Autodesk Fusion 360 part; units mm, degrees
(part 8 of 15)
  spline S126 degree 5 poles (-18.825, -121.4416) (-18.8248, -121.4521) (-18.824, -121.4806) (-18.8228, -121.5269) (-18.8208, -121.5911) (-18.818, -121.6733) (-18.8145, -121.7628) (-18.8106, -121.8524) (-18.8063, -121.942) (-18.8015, -122.0317) (-18.7964, -122.1214) (-18.7909, -122.2111) (-18.785, -122.3009) (-18.7788, -122.3908) (-18.7721, -122.4807) (-18.7651, -122.5706) (-18.7577, -122.6606) (-18.7499, -122.7506) (-18.7418, -122.8406) (-18.7333, -122.9307) (-18.7245, -123.0208) (-18.7153, -123.111) (-18.7057, -123.2012) (-18.6959, -123.2914) (-18.6856, -123.3816) (-18.6751, -123.4719) (-18.6641, -123.5622) (-18.6529, -123.6525) (-18.6413, -123.7428) (-18.6294, -123.8332) (-18.6172, -123.9236) (-18.6046, -124.014) (-18.5918, -124.1045) (-18.5786, -124.1949) (-18.565, -124.2854) (-18.5512, -124.3759) (-18.537, -124.4664) (-18.5226, -124.557) (-18.5078, -124.6475) (-18.4927, -124.7381) (-18.4774, -124.8287) (-18.4617, -124.9193) (-18.4457, -125.0099) (-18.4326, -125.0824) (-18.4227, -125.1368) (-18.4161, -125.1731) (-18.4127, -125.1912) knots 0.405839 0.405839 0.405839 0.405839 0.405839 0.405839 0.414286 0.428571 0.442857 0.457143 0.471429 0.485714 0.5 0.514286 0.528571 0.542857 0.557143 0.571429 0.585714 0.6 0.614286 0.628571 0.642857 0.657143 0.671429 0.685714 0.7 0.714286 0.728571 0.742857 0.757143 0.771429 0.785714 0.8 0.814286 0.828571 0.842857 0.857143 0.871429 0.885714 0.9 0.914286 0.928571 0.942857 0.957143 0.971429 0.985714 1 1 1 1 1 1
  arc A127 (-18.4127, -125.1912) -> (-17.1202, -125.4724) centre (-2.0032, -52.8695) ccw
  spline S127 degree 5 poles (-17.1202, -125.4724) (-17.1096, -125.4573) (-17.0884, -125.4271) (-17.0568, -125.3817) (-17.0149, -125.3212) (-16.9627, -125.2454) (-16.9108, -125.1695) (-16.8591, -125.0935) (-16.8078, -125.0174) (-16.7567, -124.9411) (-16.706, -124.8648) (-16.6555, -124.7883) (-16.6053, -124.7117) (-16.5554, -124.635) (-16.5058, -124.5582) (-16.4565, -124.4813) (-16.4076, -124.4043) (-16.3589, -124.3271) (-16.3105, -124.2499) (-16.2624, -124.1725) (-16.2147, -124.095) (-16.1673, -124.0174) (-16.1202, -123.9397) (-16.0734, -123.8618) (-16.0269, -123.7839) (-15.9808, -123.7058) (-15.9349, -123.6277) (-15.8895, -123.5494) (-15.8443, -123.4709) (-15.7995, -123.3924) (-15.7551, -123.3138) (-15.711, -123.235) (-15.6672, -123.1561) (-15.6238, -123.0771) (-15.5808, -122.998) (-15.5381, -122.9187) (-15.4958, -122.8394) (-15.4539, -122.7599) (-15.4124, -122.6803) (-15.3712, -122.6005) (-15.3305, -122.5207) (-15.2901, -122.4407) (-15.2534, -122.3672) (-15.2249, -122.3096) (-15.2045, -122.2679) (-15.1921, -122.2424) (-15.1874, -122.2329) knots -1 -1 -1 -1 -1 -1 -0.985714 -0.971429 -0.957143 -0.942857 -0.928571 -0.914286 -0.9 -0.885714 -0.871429 -0.857143 -0.842857 -0.828571 -0.814286 -0.8 -0.785714 -0.771429 -0.757143 -0.742857 -0.728571 -0.714286 -0.7 -0.685714 -0.671429 -0.657143 -0.642857 -0.628571 -0.614286 -0.6 -0.585714 -0.571429 -0.557143 -0.542857 -0.528571 -0.514286 -0.5 -0.485714 -0.471429 -0.457143 -0.442857 -0.428571 -0.414286 -0.405839 -0.405839 -0.405839 -0.405839 -0.405839 -0.405839
  arc A128 (-15.1874, -122.2329) -> (-13.8903, -122.4669) centre (-2.0032, -52.8695) ccw
  spline S128 degree 5 poles (-13.8903, -122.4669) (-13.8893, -122.4774) (-13.8865, -122.5057) (-13.882, -122.5519) (-13.8754, -122.6158) (-13.8667, -122.6975) (-13.8569, -122.7866) (-13.8466, -122.8756) (-13.8359, -122.9647) (-13.8248, -123.0538) (-13.8133, -123.1429) (-13.8014, -123.2321) (-13.7891, -123.3212) (-13.7764, -123.4104) (-13.7634, -123.4996) (-13.7499, -123.5888) (-13.7362, -123.678) (-13.722, -123.7672) (-13.7075, -123.8565) (-13.6926, -123.9457) (-13.6773, -124.035) (-13.6617, -124.1242) (-13.6458, -124.2135) (-13.6295, -124.3028) (-13.6128, -124.3921) (-13.5959, -124.4813) (-13.5785, -124.5706) (-13.5609, -124.6599) (-13.5429, -124.7492) (-13.5246, -124.8385) (-13.5059, -124.9278) (-13.4869, -125.0171) (-13.4676, -125.1064) (-13.448, -125.1957) (-13.4281, -125.285) (-13.4078, -125.3742) (-13.3873, -125.4635) (-13.3664, -125.5528) (-13.3452, -125.6421) (-13.3237, -125.7314) (-13.3019, -125.8206) (-13.2798, -125.9099) (-13.2573, -125.9991) (-13.2392, -126.0705) (-13.2254, -126.1241) (-13.2162, -126.1597) (-13.2115, -126.1776) knots 0.405839 0.405839 0.405839 0.405839 0.405839 0.405839 0.414286 0.428571 0.442857 0.457143 0.471429 0.485714 0.5 0.514286 0.528571 0.542857 0.557143 0.571429 0.585714 0.6 0.614286 0.628571 0.642857 0.657143 0.671429 0.685714 0.7 0.714286 0.728571 0.742857 0.757143 0.771429 0.785714 0.8 0.814286 0.828571 0.842857 0.857143 0.871429 0.885714 0.9 0.914286 0.928571 0.942857 0.957143 0.971429 0.985714 1 1 1 1 1 1
  arc A129 (-13.2115, -126.1776) -> (-11.9022, -126.3658) centre (-2.0032, -52.8695) ccw
  spline S129 degree 5 poles (-11.9022, -126.3658) (-11.8927, -126.35) (-11.8738, -126.3184) (-11.8455, -126.2709) (-11.808, -126.2075) (-11.7613, -126.1282) (-11.7149, -126.0488) (-11.6689, -125.9693) (-11.6231, -125.8897) (-11.5776, -125.81) (-11.5324, -125.7302) (-11.4875, -125.6503) (-11.4429, -125.5704) (-11.3986, -125.4903) (-11.3547, -125.4102) (-11.311, -125.3299) (-11.2676, -125.2496) (-11.2246, -125.1692) (-11.1818, -125.0887) (-11.1394, -125.0081) (-11.0973, -124.9274) (-11.0555, -124.8466) (-11.0141, -124.7657) (-10.973, -124.6847) (-10.9322, -124.6037) (-10.8917, -124.5225) (-10.8516, -124.4412) (-10.8118, -124.3599) (-10.7724, -124.2785) (-10.7333, -124.1969) (-10.6946, -124.1153) (-10.6562, -124.0336) (-10.6182, -123.9518) (-10.5806, -123.8699) (-10.5433, -123.7879) (-10.5064, -123.7058) (-10.4699, -123.6236) (-10.4337, -123.5414) (-10.398, -123.459) (-10.3626, -123.3765) (-10.3276, -123.294) (-10.2931, -123.2113) (-10.2617, -123.1353) (-10.2374, -123.0759) (-10.2201, -123.0329) (-10.2095, -123.0065) (-10.2055, -122.9967) knots -1 -1 -1 -1 -1 -1 -0.985714 -0.971429 -0.957143 -0.942857 -0.928571 -0.914286 -0.9 -0.885714 -0.871429 -0.857143 -0.842857 -0.828571 -0.814286 -0.8 -0.785714 -0.771429 -0.757143 -0.742857 -0.728571 -0.714286 -0.7 -0.685714 -0.671429 -0.657143 -0.642857 -0.628571 -0.614286 -0.6 -0.585714 -0.571429 -0.557143 -0.542857 -0.528571 -0.514286 -0.5 -0.485714 -0.471429 -0.457143 -0.442857 -0.428571 -0.414286 -0.405839 -0.405839 -0.405839 -0.405839 -0.405839 -0.405839
  arc A130 (-10.2055, -122.9967) -> (-8.895, -123.1376) centre (-2.0032, -52.8695) ccw
  spline S130 degree 5 poles (-8.895, -123.1376) (-8.8932, -123.148) (-8.8884, -123.1761) (-8.8806, -123.2217) (-8.8695, -123.285) (-8.855, -123.3659) (-8.8388, -123.454) (-8.8222, -123.5421) (-8.8052, -123.6302) (-8.7878, -123.7183) (-8.7699, -123.8064) (-8.7517, -123.8945) (-8.7331, -123.9825) (-8.7141, -124.0706) (-8.6947, -124.1586) (-8.675, -124.2466) (-8.6548, -124.3346) (-8.6343, -124.4226) (-8.6135, -124.5106) (-8.5923, -124.5985) (-8.5707, -124.6865) (-8.5488, -124.7744) (-8.5265, -124.8623) (-8.5039, -124.9502) (-8.4809, -125.038) (-8.4576, -125.1259) (-8.4339, -125.2137) (-8.41, -125.3015) (-8.3856, -125.3893) (-8.361, -125.4771) (-8.336, -125.5648) (-8.3107, -125.6525) (-8.2851, -125.7402) (-8.2592, -125.8279) (-8.2329, -125.9155) (-8.2063, -126.0031) (-8.1794, -126.0907) (-8.1522, -126.1783) (-8.1247, -126.2658) (-8.0969, -126.3533) (-8.0688, -126.4408) (-8.0404, -126.5282) (-8.0117, -126.6157) (-7.9884, -126.6856) (-7.9709, -126.738) (-7.9591, -126.7729) (-7.9532, -126.7904) knots 0.405839 0.405839 0.405839 0.405839 0.405839 0.405839 0.414286 0.428571 0.442857 0.457143 0.471429 0.485714 0.5 0.514286 0.528571 0.542857 0.557143 0.571429 0.585714 0.6 0.614286 0.628571 0.642857 0.657143 0.671429 0.685714 0.7 0.714286 0.728571 0.742857 0.757143 0.771429 0.785714 0.8 0.814286 0.828571 0.842857 0.857143 0.871429 0.885714 0.9 0.914286 0.928571 0.942857 0.957143 0.971429 0.985714 1 1 1 1 1 1
  arc A131 (-7.9532, -126.7904) -> (-6.6338, -126.8848) centre (-2.0032, -52.8695) ccw
  spline S131 degree 5 poles (-6.6338, -126.8848) (-6.6255, -126.8683) (-6.6089, -126.8354) (-6.584, -126.786) (-6.5511, -126.7201) (-6.5102, -126.6377) (-6.4697, -126.5552) (-6.4294, -126.4726) (-6.3894, -126.3899) (-6.3497, -126.3072) (-6.3103, -126.2244) (-6.2712, -126.1415) (-6.2325, -126.0586) (-6.194, -125.9756) (-6.1558, -125.8925) (-6.118, -125.8093) (-6.0805, -125.7261) (-6.0433, -125.6428) (-6.0064, -125.5595) (-5.9698, -125.476) (-5.9336, -125.3925) (-5.8977, -125.309) (-5.8621, -125.2253) (-5.8269, -125.1416) (-5.792, -125.0579) (-5.7574, -124.974) (-5.7232, -124.8901) (-5.6893, -124.8062) (-5.6558, -124.7221) (-5.6227, -124.638) (-5.5898, -124.5538) (-5.5574, -124.4696) (-5.5253, -124.3853) (-5.4936, -124.3009) (-5.4623, -124.2165) (-5.4313, -124.132) (-5.4008, -124.0474) (-5.3706, -123.9627) (-5.3408, -123.878) (-5.3114, -123.7932) (-5.2824, -123.7084) (-5.2538, -123.6235) (-5.228, -123.5455) (-5.208, -123.4844) (-5.1937, -123.4403) (-5.185, -123.4132) (-5.1818, -123.4032) knots -1 -1 -1 -1 -1 -1 -0.985714 -0.971429 -0.957143 -0.942857 -0.928571 -0.914286 -0.9 -0.885714 -0.871429 -0.857143 -0.842857 -0.828571 -0.814286 -0.8 -0.785714 -0.771429 -0.757143 -0.742857 -0.728571 -0.714286 -0.7 -0.685714 -0.671429 -0.657143 -0.642857 -0.628571 -0.614286 -0.6 -0.585714 -0.571429 -0.557143 -0.542857 -0.528571 -0.514286 -0.5 -0.485714 -0.471429 -0.457143 -0.442857 -0.428571 -0.414286 -0.405839 -0.405839 -0.405839 -0.405839 -0.405839 -0.405839
  arc A132 (-5.1818, -123.4032) -> (-3.8645, -123.4502) centre (-2.0032, -52.8695) ccw
  spline S132 degree 5 poles (-3.8645, -123.4502) (-3.862, -123.4605) (-3.8553, -123.4881) (-3.8442, -123.5331) (-3.8287, -123.5954) (-3.8084, -123.6751) (-3.786, -123.7619) (-3.7631, -123.8485) (-3.7398, -123.9352) (-3.7162, -124.0218) (-3.6921, -124.1084) (-3.6676, -124.1949) (-3.6428, -124.2814) (-3.6176, -124.3679) (-3.592, -124.4543) (-3.566, -124.5407) (-3.5396, -124.6271) (-3.5129, -124.7134) (-3.4858, -124.7996) (-3.4584, -124.8858) (-3.4306, -124.972) (-3.4025, -125.0581) (-3.374, -125.1442) (-3.3451, -125.2303) (-3.316, -125.3163) (-3.2864, -125.4022) (-3.2566, -125.4881) (-3.2264, -125.574) (-3.1959, -125.6598) (-3.165, -125.7456) (-3.1339, -125.8313) (-3.1024, -125.917) (-3.0706, -126.0027) (-3.0384, -126.0883) (-3.006, -126.1738) (-2.9732, -126.2593) (-2.9402, -126.3447) (-2.9068, -126.4301) (-2.8731, -126.5155) (-2.8391, -126.6008) (-2.8048, -126.686) (-2.7702, -126.7712) (-2.7354, -126.8564) (-2.7072, -126.9245) (-2.686, -126.9755) (-2.6717, -127.0095) (-2.6646, -127.0265) knots 0.405839 0.405839 0.405839 0.405839 0.405839 0.405839 0.414286 0.428571 0.442857 0.457143 0.471429 0.485714 0.5 0.514286 0.528571 0.542857 0.557143 0.571429 0.585714 0.6 0.614286 0.628571 0.642857 0.657143 0.671429 0.685714 0.7 0.714286 0.728571 0.742857 0.757143 0.771429 0.785714 0.8 0.814286 0.828571 0.842857 0.857143 0.871429 0.885714 0.9 0.914286 0.928571 0.942857 0.957143 0.971429 0.985714 1 1 1 1 1 1
  arc A133 (-2.6646, -127.0265) -> (-1.3418, -127.0265) centre (-2.0032, -52.8695) ccw
  spline S133 degree 5 poles (-1.3418, -127.0265) (-1.3347, -127.0095) (-1.3205, -126.9755) (-1.2992, -126.9245) (-1.2711, -126.8564) (-1.2362, -126.7712) (-1.2016, -126.686) (-1.1673, -126.6008) (-1.1333, -126.5155) (-1.0996, -126.4301) (-1.0663, -126.3447) (-1.0332, -126.2593) (-1.0004, -126.1738) (-0.968, -126.0883) (-0.9359, -126.0027) (-0.904, -125.917) (-0.8726, -125.8313) (-0.8414, -125.7456) (-0.8105, -125.6598) (-0.78, -125.574) (-0.7498, -125.4881) (-0.72, -125.4022) (-0.6905, -125.3163) (-0.6613, -125.2303) (-0.6325, -125.1442) (-0.604, -125.0581) (-0.5758, -124.972) (-0.548, -124.8858) (-0.5206, -124.7996) (-0.4935, -124.7134) (-0.4668, -124.6271) (-0.4405, -124.5407) (-0.4145, -124.4543) (-0.3889, -124.3679) (-0.3636, -124.2814) (-0.3388, -124.1949) (-0.3143, -124.1084) (-0.2903, -124.0218) (-0.2666, -123.9352) (-0.2433, -123.8485) (-0.2205, -123.7619) (-0.198, -123.6751) (-0.1778, -123.5954) (-0.1622, -123.5331) (-0.1511, -123.4881) (-0.1444, -123.4605) (-0.1419, -123.4502) knots -1 -1 -1 -1 -1 -1 -0.985714 -0.971429 -0.957143 -0.942857 -0.928571 -0.914286 -0.9 -0.885714 -0.871429 -0.857143 -0.842857 -0.828571 -0.814286 -0.8 -0.785714 -0.771429 -0.757143 -0.742857 -0.728571 -0.714286 -0.7 -0.685714 -0.671429 -0.657143 -0.642857 -0.628571 -0.614286 -0.6 -0.585714 -0.571429 -0.557143 -0.542857 -0.528571 -0.514286 -0.5 -0.485714 -0.471429 -0.457143 -0.442857 -0.428571 -0.414286 -0.405839 -0.405839 -0.405839 -0.405839 -0.405839 -0.405839
  arc A134 (-0.1419, -123.4502) -> (1.1754, -123.4032) centre (-2.0032, -52.8695) ccw
  spline S134 degree 5 poles (1.1754, -123.4032) (1.1786, -123.4132) (1.1873, -123.4403) (1.2016, -123.4844) (1.2215, -123.5455) (1.2474, -123.6235) (1.276, -123.7084) (1.305, -123.7932) (1.3344, -123.878) (1.3641, -123.9627) (1.3943, -124.0474) (1.4249, -124.132) (1.4559, -124.2165) (1.4872, -124.3009) (1.5189, -124.3853) (1.551, -124.4696) (1.5834, -124.5538) (1.6162, -124.638) (1.6494, -124.7221) (1.6829, -124.8062) (1.7168, -124.8901) (1.751, -124.974) (1.7855, -125.0579) (1.8205, -125.1416) (1.8557, -125.2253) (1.8913, -125.309) (1.9272, -125.3925) (1.9634, -125.476) (2, -125.5595) (2.0368, -125.6428) (2.074, -125.7261) (2.1116, -125.8093) (2.1494, -125.8925) (2.1876, -125.9756) (2.226, -126.0586) (2.2648, -126.1415) (2.3039, -126.2244) (2.3433, -126.3072) (2.383, -126.3899) (2.4229, -126.4726) (2.4632, -126.5552) (2.5038, -126.6377) (2.5447, -126.7201) (2.5776, -126.786) (2.6024, -126.8354) (2.6191, -126.8683) (2.6274, -126.8848) knots 0.405839 0.405839 0.405839 0.405839 0.405839 0.405839 0.414286 0.428571 0.442857 0.457143 0.471429 0.485714 0.5 0.514286 0.528571 0.542857 0.557143 0.571429 0.585714 0.6 0.614286 0.628571 0.642857 0.657143 0.671429 0.685714 0.7 0.714286 0.728571 0.742857 0.757143 0.771429 0.785714 0.8 0.814286 0.828571 0.842857 0.857143 0.871429 0.885714 0.9 0.914286 0.928571 0.942857 0.957143 0.971429 0.985714 1 1 1 1 1 1
  arc A135 (2.6274, -126.8848) -> (3.9468, -126.7904) centre (-2.0032, -52.8695) ccw
  spline S135 degree 5 poles (3.9468, -126.7904) (3.9527, -126.7729) (3.9645, -126.738) (3.982, -126.6856) (4.0052, -126.6157) (4.034, -126.5282) (4.0624, -126.4408) (4.0905, -126.3533) (4.1183, -126.2658) (4.1458, -126.1783) (4.173, -126.0907) (4.1999, -126.0031) (4.2265, -125.9155) (4.2527, -125.8279) (4.2787, -125.7402) (4.3043, -125.6525) (4.3296, -125.5648) (4.3546, -125.4771) (4.3792, -125.3893) (4.4035, -125.3015) (4.4275, -125.2137) (4.4512, -125.1259) (4.4745, -125.038) (4.4974, -124.9502) (4.5201, -124.8623) (4.5423, -124.7744) (4.5643, -124.6865) (4.5858, -124.5985) (4.6071, -124.5106) (4.6279, -124.4226) (4.6484, -124.3346) (4.6685, -124.2466) (4.6883, -124.1586) (4.7077, -124.0706) (4.7267, -123.9825) (4.7453, -123.8945) (4.7635, -123.8064) (4.7813, -123.7183) (4.7988, -123.6302) (4.8158, -123.5421) (4.8324, -123.454) (4.8486, -123.3659) (4.8631, -123.285) (4.8742, -123.2217) (4.882, -123.1761) (4.8868, -123.148) (4.8885, -123.1376) knots -1 -1 -1 -1 -1 -1 -0.985714 -0.971429 -0.957143 -0.942857 -0.928571 -0.914286 -0.9 -0.885714 -0.871429 -0.857143 -0.842857 -0.828571 -0.814286 -0.8 -0.785714 -0.771429 -0.757143 -0.742857 -0.728571 -0.714286 -0.7 -0.685714 -0.671429 -0.657143 -0.642857 -0.628571 -0.614286 -0.6 -0.585714 -0.571429 -0.557143 -0.542857 -0.528571 -0.514286 -0.5 -0.485714 -0.471429 -0.457143 -0.442857 -0.428571 -0.414286 -0.405839 -0.405839 -0.405839 -0.405839 -0.405839 -0.405839
  arc A136 (4.8885, -123.1376) -> (6.1991, -122.9967) centre (-2.0032, -52.8695) ccw
  spline S136 degree 5 poles (6.1991, -122.9967) (6.203, -123.0065) (6.2136, -123.0329) (6.231, -123.0759) (6.2553, -123.1353) (6.2866, -123.2113) (6.3212, -123.294) (6.3562, -123.3765) (6.3915, -123.459) (6.4273, -123.5414) (6.4634, -123.6236) (6.5, -123.7058) (6.5369, -123.7879) (6.5742, -123.8699) (6.6118, -123.9518) (6.6498, -124.0336) (6.6882, -124.1153) (6.7269, -124.1969) (6.766, -124.2785) (6.8054, -124.3599) (6.8452, -124.4412) (6.8853, -124.5225) (6.9258, -124.6037) (6.9665, -124.6847) (7.0077, -124.7657) (7.0491, -124.8466) (7.0909, -124.9274) (7.133, -125.0081) (7.1754, -125.0887) (7.2181, -125.1692) (7.2612, -125.2496) (7.3046, -125.3299) (7.3482, -125.4102) (7.3922, -125.4903) (7.4365, -125.5704) (7.4811, -125.6503) (7.526, -125.7302) (7.5712, -125.81) (7.6167, -125.8897) (7.6624, -125.9693) (7.7085, -126.0488) (7.7549, -126.1282) (7.8015, -126.2075) (7.8391, -126.2709) (7.8674, -126.3184) (7.8863, -126.35) (7.8958, -126.3658) knots 0.405839 0.405839 0.405839 0.405839 0.405839 0.405839 0.414286 0.428571 0.442857 0.457143 0.471429 0.485714 0.5 0.514286 0.528571 0.542857 0.557143 0.571429 0.585714 0.6 0.614286 0.628571 0.642857 0.657143 0.671429 0.685714 0.7 0.714286 0.728571 0.742857 0.757143 0.771429 0.785714 0.8 0.814286 0.828571 0.842857 0.857143 0.871429 0.885714 0.9 0.914286 0.928571 0.942857 0.957143 0.971429 0.985714 1 1 1 1 1 1
  arc A137 (7.8958, -126.3658) -> (9.2051, -126.1776) centre (-2.0032, -52.8695) ccw
  spline S137 degree 5 poles (9.2051, -126.1776) (9.2097, -126.1597) (9.219, -126.1241) (9.2327, -126.0705) (9.2509, -125.9991) (9.2733, -125.9099) (9.2954, -125.8206) (9.3172, -125.7314) (9.3387, -125.6421) (9.3599, -125.5528) (9.3808, -125.4635) (9.4014, -125.3742) (9.4217, -125.285) (9.4416, -125.1957) (9.4612, -125.1064) (9.4805, -125.0171) (9.4995, -124.9278) (9.5181, -124.8385) (9.5365, -124.7492) (9.5545, -124.6599) (9.5721, -124.5706) (9.5894, -124.4813) (9.6064, -124.3921) (9.6231, -124.3028) (9.6394, -124.2135) (9.6553, -124.1242) (9.6709, -124.035) (9.6861, -123.9457) (9.701, -123.8565) (9.7156, -123.7672) (9.7297, -123.678) (9.7435, -123.5888) (9.7569, -123.4996) (9.77, -123.4104) (9.7827, -123.3212) (9.7949, -123.2321) (9.8068, -123.1429) (9.8183, -123.0538) (9.8294, -122.9647) (9.8401, -122.8756) (9.8504, -122.7866) (9.8603, -122.6975) (9.869, -122.6158) (9.8755, -122.5519) (9.8801, -122.5057) (9.8828, -122.4774) (9.8838, -122.4669) knots -1 -1 -1 -1 -1 -1 -0.985714 -0.971429 -0.957143 -0.942857 -0.928571 -0.914286 -0.9 -0.885714 -0.871429 -0.857143 -0.842857 -0.828571 -0.814286 -0.8 -0.785714 -0.771429 -0.757143 -0.742857 -0.728571 -0.714286 -0.7 -0.685714 -0.671429 -0.657143 -0.642857 -0.628571 -0.614286 -0.6 -0.585714 -0.571429 -0.557143 -0.542857 -0.528571 -0.514286 -0.5 -0.485714 -0.471429 -0.457143 -0.442857 -0.428571 -0.414286 -0.405839 -0.405839 -0.405839 -0.405839 -0.405839 -0.405839
  arc A138 (9.8838, -122.4669) -> (11.181, -122.2329) centre (-2.0032, -52.8695) ccw
  spline S138 degree 5 poles (11.181, -122.2329) (11.1856, -122.2424) (11.1981, -122.2679) (11.2185, -122.3096) (11.2469, -122.3672) (11.2837, -122.4407) (11.324, -122.5207) (11.3648, -122.6005) (11.406, -122.6803) (11.4475, -122.7599) (11.4894, -122.8394) (11.5317, -122.9187) (11.5744, -122.998) (11.6174, -123.0771) (11.6608, -123.1561) (11.7046, -123.235) (11.7487, -123.3138) (11.7931, -123.3924) (11.8379, -123.4709) (11.883, -123.5494) (11.9285, -123.6277) (11.9743, -123.7058) (12.0205, -123.7839) (12.0669, -123.8618) (12.1137, -123.9397) (12.1608, -124.0174) (12.2083, -124.095) (12.256, -124.1725) (12.3041, -124.2499) (12.3524, -124.3271) (12.4011, -124.4043) (12.4501, -124.4813) (12.4994, -124.5582) (12.549, -124.635) (12.5989, -124.7117) (12.6491, -124.7883) (12.6995, -124.8648) (12.7503, -124.9411) (12.8014, -125.0174) (12.8527, -125.0935) (12.9043, -125.1695) (12.9562, -125.2454) (13.0084, -125.3212) (13.0504, -125.3817) (13.082, -125.4271) (13.1031, -125.4573) (13.1137, -125.4724) knots 0.405839 0.405839 0.405839 0.405839 0.405839 0.405839 0.414286 0.428571 0.442857 0.457143 0.471429 0.485714 0.5 0.514286 0.528571 0.542857 0.557143 0.571429 0.585714 0.6 0.614286 0.628571 0.642857 0.657143 0.671429 0.685714 0.7 0.714286 0.728571 0.742857 0.757143 0.771429 0.785714 0.8 0.814286 0.828571 0.842857 0.857143 0.871429 0.885714 0.9 0.914286 0.928571 0.942857 0.957143 0.971429 0.985714 1 1 1 1 1 1
  arc A139 (13.1137, -125.4724) -> (14.4063, -125.1912) centre (-2.0032, -52.8695) ccw
  spline S139 degree 5 poles (14.4063, -125.1912) (14.4096, -125.1731) (14.4163, -125.1368) (14.4262, -125.0824) (14.4392, -125.0099) (14.4552, -124.9193) (14.4709, -124.8287) (14.4863, -124.7381) (14.5014, -124.6475) (14.5162, -124.557) (14.5306, -124.4664) (14.5448, -124.3759) (14.5586, -124.2854) (14.5721, -124.1949) (14.5853, -124.1045) (14.5982, -124.014) (14.6108, -123.9236) (14.623, -123.8332) (14.6349, -123.7428) (14.6465, -123.6525) (14.6577, -123.5622) (14.6686, -123.4719) (14.6792, -123.3816) (14.6894, -123.2914) (14.6993, -123.2012) (14.7089, -123.111) (14.718, -123.0208) (14.7269, -122.9307) (14.7354, -122.8406) (14.7435, -122.7506) (14.7513, -122.6606) (14.7586, -122.5706) (14.7657, -122.4807) (14.7723, -122.3908) (14.7786, -122.3009) (14.7845, -122.2111) (14.79, -122.1214) (14.7951, -122.0317) (14.7998, -121.942) (14.8041, -121.8524) (14.8081, -121.7628) (14.8116, -121.6733) (14.8144, -121.5911) (14.8163, -121.5269) (14.8176, -121.4806) (14.8183, -121.4521) (14.8186, -121.4416) knots -1 -1 -1 -1 -1 -1 -0.985714 -0.971429 -0.957143 -0.942857 -0.928571 -0.914286 -0.9 -0.885714 -0.871429 -0.857143 -0.842857 -0.828571 -0.814286 -0.8 -0.785714 -0.771429 -0.757143 -0.742857 -0.728571 -0.714286 -0.7 -0.685714 -0.671429 -0.657143 -0.642857 -0.628571 -0.614286 -0.6 -0.585714 -0.571429 -0.557143 -0.542857 -0.528571 -0.514286 -0.5 -0.485714 -0.471429 -0.457143 -0.442857 -0.428571 -0.414286 -0.405839 -0.405839 -0.405839 -0.405839 -0.405839 -0.405839
  arc A140 (14.8186, -121.4416) -> (16.0958, -121.1156) centre (-2.0032, -52.8695) ccw
  spline S140 degree 5 poles (16.0958, -121.1156) (16.101, -121.1247) (16.1153, -121.1493) (16.1386, -121.1894) (16.1711, -121.2448) (16.213, -121.3156) (16.2589, -121.3925) (16.3053, -121.4692) (16.352, -121.5458) (16.3991, -121.6222) (16.4466, -121.6985) (16.4945, -121.7747) (16.5427, -121.8507) (16.5913, -121.9265) (16.6402, -122.0022) (16.6895, -122.0778) (16.7391, -122.1532) (16.789, -122.2285) (16.8393, -122.3036) (16.8899, -122.3786) (16.9409, -122.4535) (16.9921, -122.5282) (17.0437, -122.6028) (17.0956, -122.6772) (17.1478, -122.7515) (17.2004, -122.8257) (17.2532, -122.8997) (17.3064, -122.9736) (17.3598, -123.0473) (17.4136, -123.1209) (17.4677, -123.1944) (17.522, -123.2678) (17.5767, -123.341) (17.6316, -123.414) (17.6868, -123.487) (17.7424, -123.5598) (17.7982, -123.6325) (17.8542, -123.705) (17.9106, -123.7774) (17.9672, -123.8497) (18.0242, -123.9218) (18.0814, -123.9938) (18.1388, -124.0657) (18.185, -124.1231) (18.2198, -124.166) (18.243, -124.1947) (18.2546, -124.209) knots 0.405839 0.405839 0.405839 0.405839 0.405839 0.405839 0.414286 0.428571 0.442857 0.457143 0.471429 0.485714 0.5 0.514286 0.528571 0.542857 0.557143 0.571429 0.585714 0.6 0.614286 0.628571 0.642857 0.657143 0.671429 0.685714 0.7 0.714286 0.728571 0.742857 0.757143 0.771429 0.785714 0.8 0.814286 0.828571 0.842857 0.857143 0.871429 0.885714 0.9 0.914286 0.928571 0.942857 0.957143 0.971429 0.985714 1 1 1 1 1 1
  arc A141 (18.2546, -124.209) -> (19.5238, -123.8363) centre (-2.0032, -52.8695) ccw
  spline S141 degree 5 poles (19.5238, -123.8363) (19.5259, -123.818) (19.53, -123.7813) (19.536, -123.7264) (19.5438, -123.6531) (19.5533, -123.5616) (19.5625, -123.4701) (19.5713, -123.3787) (19.5799, -123.2872) (19.5882, -123.1959) (19.5962, -123.1045) (19.6038, -123.0132) (19.6112, -122.9219) (19.6182, -122.8307) (19.6249, -122.7396) (19.6313, -122.6484) (19.6374, -122.5573) (19.6431, -122.4663) (19.6486, -122.3753) (19.6537, -122.2844) (19.6584, -122.1935) (19.6629, -122.1026) (19.667, -122.0118) (19.6707, -121.9211) (19.6742, -121.8304) (19.6772, -121.7398) (19.68, -121.6492) (19.6824, -121.5587) (19.6844, -121.4682) (19.6861, -121.3778) (19.6874, -121.2875) (19.6884, -121.1972) (19.689, -121.107) (19.6892, -121.0169) (19.689, -120.9268) (19.6885, -120.8368) (19.6876, -120.7469) (19.6863, -120.6571) (19.6846, -120.5673) (19.6825, -120.4776) (19.68, -120.388) (19.6771, -120.2984) (19.6741, -120.2163) (19.6715, -120.1521) (19.6694, -120.1058) (19.6681, -120.0774) (19.6676, -120.0668) knots -1 -1 -1 -1 -1 -1 -0.985714 -0.971429 -0.957143 -0.942857 -0.928571 -0.914286 -0.9 -0.885714 -0.871429 -0.857143 -0.842857 -0.828571 -0.814286 -0.8 -0.785714 -0.771429 -0.757143 -0.742857 -0.728571 -0.714286 -0.7 -0.685714 -0.671429 -0.657143 -0.642857 -0.628571 -0.614286 -0.6 -0.585714 -0.571429 -0.557143 -0.542857 -0.528571 -0.514286 -0.5 -0.485714 -0.471429 -0.457143 -0.442857 -0.428571 -0.414286 -0.405839 -0.405839 -0.405839 -0.405839 -0.405839 -0.405839
  arc A142 (19.6676, -120.0668) -> (20.9183, -119.6505) centre (-2.0032, -52.8695) ccw
  spline S142 degree 5 poles (20.9183, -119.6505) (20.9242, -119.6593) (20.9402, -119.6828) (20.9663, -119.7211) (21.0026, -119.7741) (21.0494, -119.8417) (21.1008, -119.9151) (21.1525, -119.9883) (21.2046, -120.0614) (21.257, -120.1343) (21.3098, -120.207) (21.363, -120.2795) (21.4165, -120.3519) (21.4704, -120.4241) (21.5246, -120.4961) (21.5791, -120.5679) (21.634, -120.6396) (21.6891, -120.7112) (21.7447, -120.7825) (21.8005, -120.8537) (21.8566, -120.9247) (21.9131, -120.9956) (21.9699, -121.0663) (22.027, -121.1369) (22.0844, -121.2072) (22.1421, -121.2775) (22.2001, -121.3475) (22.2584, -121.4174) (22.3169, -121.4872) (22.3758, -121.5568) (22.435, -121.6262) (22.4944, -121.6955) (22.5542, -121.7646) (22.6142, -121.8336) (22.6745, -121.9024) (22.735, -121.971) (22.7959, -122.0395) (22.857, -122.1079) (22.9184, -122.1761) (22.98, -122.2441) (23.042, -122.312) (23.1041, -122.3798) (23.1666, -122.4474) (23.2168, -122.5013) (23.2545, -122.5417) (23.2797, -122.5686) (23.2923, -122.582) knots 0.405839 0.405839 0.405839 0.405839 0.405839 0.405839 0.414286 0.428571 0.442857 0.457143 0.471429 0.485714 0.5 0.514286 0.528571 0.542857 0.557143 0.571429 0.585714 0.6 0.614286 0.628571 0.642857 0.657143 0.671429 0.685714 0.7 0.714286 0.728571 0.742857 0.757143 0.771429 0.785714 0.8 0.814286 0.828571 0.842857 0.857143 0.871429 0.885714 0.9 0.914286 0.928571 0.942857 0.957143 0.971429 0.985714 1 1 1 1 1 1
  arc A143 (23.2923, -122.582) -> (24.5317, -122.1198) centre (-2.0032, -52.8695) ccw
  spline S143 degree 5 poles (24.5317, -122.1198) (24.5324, -122.1014) (24.5339, -122.0645) (24.536, -122.0093) (24.5385, -121.9356) (24.5415, -121.8437) (24.5441, -121.7518) (24.5464, -121.6599) (24.5485, -121.5681) (24.5502, -121.4764) (24.5516, -121.3847) (24.5528, -121.2931) (24.5536, -121.2015) (24.5541, -121.11) (24.5543, -121.0186) (24.5542, -120.9272) (24.5537, -120.836) (24.553, -120.7447) (24.5519, -120.6536) (24.5505, -120.5625) (24.5488, -120.4715) (24.5467, -120.3806) (24.5443, -120.2897) (24.5416, -120.199) (24.5385, -120.1083) (24.5352, -120.0176) (24.5314, -119.9271) (24.5273, -119.8366) (24.5229, -119.7463) (24.5182, -119.656) (24.513, -119.5658) (24.5075, -119.4757) (24.5017, -119.3857) (24.4955, -119.2958) (24.4889, -119.2059) (24.482, -119.1162) (24.4746, -119.0266) (24.4669, -118.937) (24.4588, -118.8476) (24.4504, -118.7583) (24.4415, -118.6691) (24.4322, -118.58) (24.4233, -118.4982) (24.4161, -118.4344) (24.4108, -118.3884) (24.4074, -118.3601) (24.4062, -118.3496) knots -1 -1 -1 -1 -1 -1 -0.985714 -0.971429 -0.957143 -0.942857 -0.928571 -0.914286 -0.9 -0.885714 -0.871429 -0.857143 -0.842857 -0.828571 -0.814286 -0.8 -0.785714 -0.771429 -0.757143 -0.742857 -0.728571 -0.714286 -0.7 -0.685714 -0.671429 -0.657143 -0.642857 -0.628571 -0.614286 -0.6 -0.585714 -0.571429 -0.557143 -0.542857 -0.528571 -0.514286 -0.5 -0.485714 -0.471429 -0.457143 -0.442857 -0.428571 -0.414286 -0.405839 -0.405839 -0.405839 -0.405839 -0.405839 -0.405839
  arc A144 (24.4062, -118.3496) -> (25.624, -117.8452) centre (-2.0032, -52.8695) ccw
  spline S144 degree 5 poles (25.624, -117.8452) (25.6305, -117.8535) (25.6481, -117.8758) (25.6769, -117.9122) (25.7169, -117.9624) (25.7684, -118.0265) (25.8249, -118.096) (25.8817, -118.1654) (25.9389, -118.2346) (25.9964, -118.3035) (26.0542, -118.3723) (26.1124, -118.4408) (26.171, -118.5092) (26.2298, -118.5774) (26.289, -118.6453) (26.3486, -118.7131) (26.4084, -118.7807) (26.4685, -118.8481) (26.529, -118.9153) (26.5898, -118.9824) (26.6509, -119.0492) (26.7122, -119.1159) (26.7739, -119.1823) (26.8359, -119.2486) (26.8982, -119.3147) (26.9607, -119.3807) (27.0236, -119.4464) (27.0867, -119.512) (27.1501, -119.5774) (27.2138, -119.6426) (27.2778, -119.7076) (27.342, -119.7725) (27.4065, -119.8372) (27.4713, -119.9017) (27.5363, -119.966) (27.6017, -120.0302) (27.6672, -120.0942) (27.7331, -120.158) (27.7992, -120.2216) (27.8655, -120.2851) (27.9321, -120.3484) (27.999, -120.4115) (28.0661, -120.4745) (28.12, -120.5247) (28.1605, -120.5623) (28.1876, -120.5873) (28.2011, -120.5999) knots 0.405839 0.405839 0.405839 0.405839 0.405839 0.405839 0.414286 0.428571 0.442857 0.457143 0.471429 0.485714 0.5 0.514286 0.528571 0.542857 0.557143 0.571429 0.585714 0.6 0.614286 0.628571 0.642857 0.657143 0.671429 0.685714 0.7 0.714286 0.728571 0.742857 0.757143 0.771429 0.785714 0.8 0.814286 0.828571 0.842857 0.857143 0.871429 0.885714 0.9 0.914286 0.928571 0.942857 0.957143 0.971429 0.985714 1 1 1 1 1 1
  arc A145 (28.2011, -120.5999) -> (29.4044, -120.0504) centre (-2.0032, -52.8695) ccw
  spline S145 degree 5 poles (29.4044, -120.0504) (29.4038, -120.0319) (29.4026, -119.9951) (29.4007, -119.9398) (29.398, -119.8662) (29.3944, -119.7743) (29.3905, -119.6824) (29.3862, -119.5906) (29.3817, -119.4989) (29.3769, -119.4073) (29.3718, -119.3157) (29.3664, -119.2242) (29.3607, -119.1329) (29.3546, -119.0416) (29.3483, -118.9504) (29.3417, -118.8593) (29.3347, -118.7682) (29.3275, -118.6773) (29.3199, -118.5865) (29.312, -118.4957) (29.3038, -118.4051) (29.2952, -118.3145) (29.2864, -118.2241) (29.2772, -118.1337) (29.2677, -118.0435) (29.2578, -117.9533) (29.2477, -117.8633) (29.2371, -117.7734) (29.2263, -117.6835) (29.2151, -117.5938) (29.2035, -117.5042) (29.1916, -117.4147) (29.1794, -117.3254) (29.1668, -117.2361) (29.1538, -117.147) (29.1405, -117.058) (29.1268, -116.9691) (29.1127, -116.8803) (29.0982, -116.7917) (29.0834, -116.7032) (29.0682, -116.6149) (29.0526, -116.5266) (29.0379, -116.4458) (29.0261, -116.3826) (29.0175, -116.3371) (29.0122, -116.3091) (29.0102, -116.2987) knots -1 -1 -1 -1 -1 -1 -0.985714 -0.971429 -0.957143 -0.942857 -0.928571 -0.914286 -0.9 -0.885714 -0.871429 -0.857143 -0.842857 -0.828571 -0.814286 -0.8 -0.785714 -0.771429 -0.757143 -0.742857 -0.728571 -0.714286 -0.7 -0.685714 -0.671429 -0.657143 -0.642857 -0.628571 -0.614286 -0.6 -0.585714 -0.571429 -0.557143 -0.542857 -0.528571 -0.514286 -0.5 -0.485714 -0.471429 -0.457143 -0.442857 -0.428571 -0.414286 -0.405839 -0.405839 -0.405839 -0.405839 -0.405839 -0.405839
  arc A146 (29.0102, -116.2987) -> (30.1889, -115.7087) centre (-2.0032, -52.8695) ccw
  spline S146 degree 5 poles (30.1889, -115.7087) (30.196, -115.7166) (30.2152, -115.7376) (30.2465, -115.7718) (30.29, -115.819) (30.3459, -115.8792) (30.4072, -115.9446) (30.4688, -116.0097) (30.5308, -116.0746) (30.593, -116.1393) (30.6557, -116.2038) (30.7186, -116.268) (30.7819, -116.332) (30.8455, -116.3958) (30.9093, -116.4594) (30.9736, -116.5228) (31.0381, -116.5859) (31.1029, -116.6489) (31.168, -116.7116) (31.2334, -116.7741) (31.2991, -116.8364) (31.365, -116.8985) (31.4313, -116.9604) (31.4979, -117.0221) (31.5647, -117.0836) (31.6318, -117.1449) (31.6992, -117.206) (31.7668, -117.2669) (31.8347, -117.3276) (31.9029, -117.3881) (31.9713, -117.4484) (32.04, -117.5086) (32.109, -117.5685) (32.1782, -117.6282) (32.2477, -117.6877) (32.3174, -117.7471) (32.3874, -117.8062) (32.4576, -117.8652) (32.5281, -117.9239) (32.5988, -117.9825) (32.6697, -118.0409) (32.7409, -118.0991) (32.8124, -118.1571) (32.8697, -118.2034) (32.9128, -118.238) (32.9416, -118.261) (32.956, -118.2725) knots 0.405839 0.405839 0.405839 0.405839 0.405839 0.405839 0.414286 0.428571 0.442857 0.457143 0.471429 0.485714 0.5 0.514286 0.528571 0.542857 0.557143 0.571429 0.585714 0.6 0.614286 0.628571 0.642857 0.657143 0.671429 0.685714 0.7 0.714286 0.728571 0.742857 0.757143 0.771429 0.785714 0.8 0.814286 0.828571 0.842857 0.857143 0.871429 0.885714 0.9 0.914286 0.928571 0.942857 0.957143 0.971429 0.985714 1 1 1 1 1 1
  arc A147 (32.956, -118.2725) -> (34.117, -117.6386) centre (-2.0032, -52.8695) ccw
  spline S147 degree 5 poles (34.117, -117.6386) (34.1151, -117.6203) (34.1113, -117.5836) (34.1054, -117.5286) (34.0975, -117.4554) (34.0873, -117.3639) (34.0769, -117.2726) (34.0661, -117.1813) (34.0551, -117.0901) (34.0437, -116.9991) (34.0321, -116.9081) (34.0202, -116.8173) (34.0079, -116.7266) (33.9954, -116.6359) (33.9826, -116.5454) (33.9695, -116.455) (33.956, -116.3647) (33.9423, -116.2745) (33.9283, -116.1845) (33.9139, -116.0945) (33.8993, -116.0047) (33.8843, -115.915) (33.869, -115.8254) (33.8534, -115.7359) (33.8375, -115.6466) (33.8212, -115.5574) (33.8046, -115.4683) (33.7877, -115.3793) (33.7705, -115.2905) (33.7529, -115.2018) (33.735, -115.1133) (33.7168, -115.0249) (33.6982, -114.9366) (33.6792, -114.8485) (33.6599, -114.7605) (33.6403, -114.6727) (33.6203, -114.585) (33.5999, -114.4975) (33.5792, -114.4101) (33.5581, -114.3229) (33.5366, -114.2358) (33.5147, -114.149) (33.4943, -114.0693) (33.4781, -114.0072) (33.4662, -113.9624) (33.4589, -113.9349) (33.4562, -113.9247) knots -1 -1 -1 -1 -1 -1 -0.985714 -0.971429 -0.957143 -0.942857 -0.928571 -0.914286 -0.9 -0.885714 -0.871429 -0.857143 -0.842857 -0.828571 -0.814286 -0.8 -0.785714 -0.771429 -0.757143 -0.742857 -0.728571 -0.714286 -0.7 -0.685714 -0.671429 -0.657143 -0.642857 -0.628571 -0.614286 -0.6 -0.585714 -0.571429 -0.557143 -0.542857 -0.528571 -0.514286 -0.5 -0.485714 -0.471429 -0.457143 -0.442857 -0.428571 -0.414286 -0.405839 -0.405839 -0.405839 -0.405839 -0.405839 -0.405839
  arc A148 (33.4562, -113.9247) -> (34.5898, -113.2521) centre (-2.0032, -52.8695) ccw
  spline S148 degree 5 poles (34.5898, -113.2521) (34.5974, -113.2594) (34.618, -113.279) (34.6517, -113.3108) (34.6985, -113.3549) (34.7586, -113.4109) (34.8243, -113.4718) (34.8904, -113.5323) (34.9569, -113.5927) (35.0236, -113.6527) (35.0907, -113.7126) (35.158, -113.7721) (35.2257, -113.8315) (35.2937, -113.8906) (35.3619, -113.9494) (35.4305, -114.008) (35.4994, -114.0664) (35.5685, -114.1246) (35.6379, -114.1825) (35.7076, -114.2402) (35.7776, -114.2977) (35.8478, -114.3549) (35.9183, -114.412) (35.9891, -114.4687) (36.0601, -114.5253) (36.1314, -114.5817) (36.203, -114.6378) (36.2748, -114.6937) (36.3469, -114.7494) (36.4192, -114.8049) (36.4918, -114.8602) (36.5646, -114.9152) (36.6377, -114.9701) (36.711, -115.0247) (36.7845, -115.0791) (36.8583, -115.1334) (36.9323, -115.1874) (37.0065, -115.2412) (37.081, -115.2947) (37.1557, -115.3481) (37.2307, -115.4013) (37.3058, -115.4543) (37.3812, -115.5071) (37.4417, -115.5491) (37.4872, -115.5806) (37.5175, -115.6015) (37.5327, -115.6119) knots 0.405839 0.405839 0.405839 0.405839 0.405839 0.405839 0.414286 0.428571 0.442857 0.457143 0.471429 0.485714 0.5 0.514286 0.528571 0.542857 0.557143 0.571429 0.585714 0.6 0.614286 0.628571 0.642857 0.657143 0.671429 0.685714 0.7 0.714286 0.728571 0.742857 0.757143 0.771429 0.785714 0.8 0.814286 0.828571 0.842857 0.857143 0.871429 0.885714 0.9 0.914286 0.928571 0.942857 0.957143 0.971429 0.985714 1 1 1 1 1 1
  arc A149 (37.5327, -115.6119) -> (38.6455, -114.8968) centre (-2.0032, -52.8695) ccw
  spline S149 degree 5 poles (38.6455, -114.8968) (38.6423, -114.8786) (38.6359, -114.8423) (38.6262, -114.7879) (38.613, -114.7154) (38.5964, -114.6249) (38.5794, -114.5345) (38.5622, -114.4443) (38.5446, -114.3541) (38.5268, -114.2641) (38.5087, -114.1742) (38.4904, -114.0845) (38.4717, -113.9949) (38.4527, -113.9054) (38.4335, -113.816) (38.414, -113.7267) (38.3941, -113.6376) (38.374, -113.5487) (38.3536, -113.4598) (38.3328, -113.3711) (38.3118, -113.2826) (38.2905, -113.1942) (38.2688, -113.1059) (38.2469, -113.0178) (38.2246, -112.9298) (38.202, -112.842) (38.1791, -112.7543) (38.1559, -112.6668) (38.1324, -112.5794) (38.1085, -112.4922) (38.0844, -112.4051) (38.0599, -112.3183) (38.035, -112.2316) (38.0098, -112.145) (37.9843, -112.0586) (37.9584, -111.9724) (37.9322, -111.8864) (37.9057, -111.8005) (37.8788, -111.7149) (37.8515, -111.6294) (37.8238, -111.5441) (37.7958, -111.459) (37.7698, -111.381) (37.7492, -111.3202) (37.7342, -111.2763) (37.7249, -111.2494) (37.7214, -111.2395) knots -1 -1 -1 -1 -1 -1 -0.985714 -0.971429 -0.957143 -0.942857 -0.928571 -0.914286 -0.9 -0.885714 -0.871429 -0.857143 -0.842857 -0.828571 -0.814286 -0.8 -0.785714 -0.771429 -0.757143 -0.742857 -0.728571 -0.714286 -0.7 -0.685714 -0.671429 -0.657143 -0.642857 -0.628571 -0.614286 -0.6 -0.585714 -0.571429 -0.557143 -0.542857 -0.528571 -0.514286 -0.5 -0.485714 -0.471429 -0.457143 -0.442857 -0.428571 -0.414286 -0.405839 -0.405839 -0.405839 -0.405839 -0.405839 -0.405839
  arc A150 (37.7214, -111.2395) -> (38.8042, -110.4877) centre (-2.0032, -52.8695) ccw
  spline S150 degree 5 poles (38.8042, -110.4877) (38.8123, -110.4944) (38.8343, -110.5125) (38.8701, -110.5419) (38.9199, -110.5825) (38.9839, -110.6341) (39.0538, -110.6901) (39.1241, -110.7458) (39.1946, -110.8012) (39.2655, -110.8564) (39.3367, -110.9113) (39.4081, -110.9659) (39.4798, -111.0203) (39.5518, -111.0744) (39.6241, -111.1282) (39.6967, -111.1818) (39.7695, -111.2351) (39.8426, -111.2882) (39.916, -111.341) (39.9896, -111.3936) (40.0635, -111.4459) (40.1377, -111.498) (40.2121, -111.5499) (40.2867, -111.6015) (40.3616, -111.6528) (40.4368, -111.7039) (40.5122, -111.7548) (40.5878, -111.8055) (40.6636, -111.8559) (40.7397, -111.9061) (40.8161, -111.956) (40.8926, -112.0058) (40.9694, -112.0553) (41.0464, -112.1045) (41.1237, -112.1536) (41.2011, -112.2024) (41.2788, -112.251) (41.3567, -112.2993) (41.4348, -112.3475) (41.5131, -112.3954) (41.5917, -112.4431) (41.6704, -112.4906) (41.7494, -112.5378) (41.8127, -112.5754) (41.8603, -112.6036) (41.8921, -112.6223) (41.908, -112.6316) knots 0.405839 0.405839 0.405839 0.405839 0.405839 0.405839 0.414286 0.428571 0.442857 0.457143 0.471429 0.485714 0.5 0.514286 0.528571 0.542857 0.557143 0.571429 0.585714 0.6 0.614286 0.628571 0.642857 0.657143 0.671429 0.685714 0.7 0.714286 0.728571 0.742857 0.757143 0.771429 0.785714 0.8 0.814286 0.828571 0.842857 0.857143 0.871429 0.885714 0.9 0.914286 0.928571 0.942857 0.957143 0.971429 0.985714 1 1 1 1 1 1
  arc A151 (41.908, -112.6316) -> (42.9669, -111.8389) centre (-2.0032, -52.8695) ccw
  spline S151 degree 5 poles (42.9669, -111.8389) (42.9624, -111.821) (42.9534, -111.7853) (42.9399, -111.7317) (42.9216, -111.6603) (42.8985, -111.5712) (42.8751, -111.4823) (42.8515, -111.3935) (42.8276, -111.3048) (42.8034, -111.2163) (42.7789, -111.128) (42.7542, -111.0397) (42.7292, -110.9517) (42.7039, -110.8637) (42.6783, -110.776) (42.6525, -110.6884) (42.6263, -110.6009) (42.5999, -110.5136) (42.5732, -110.4264) (42.5462, -110.3394) (42.5189, -110.2526) (42.4913, -110.1659) (42.4634, -110.0794) (42.4353, -109.9931) (42.4068, -109.9069) (42.378, -109.8209) (42.3489, -109.7351) (42.3195, -109.6495) (42.2898, -109.564) (42.2598, -109.4787) (42.2295, -109.3936) (42.1988, -109.3087) (42.1678, -109.224) (42.1365, -109.1395) (42.1049, -109.0551) (42.073, -108.971) (42.0407, -108.8871) (42.0081, -108.8033) (41.9751, -108.7198) (41.9418, -108.6365) (41.9082, -108.5534) (41.8742, -108.4705) (41.8426, -108.3946) (41.8177, -108.3354) (41.7996, -108.2927) (41.7885, -108.2665) (41.7843, -108.2568) knots -1 -1 -1 -1 -1 -1 -0.985714 -0.971429 -0.957143 -0.942857 -0.928571 -0.914286 -0.9 -0.885714 -0.871429 -0.857143 -0.842857 -0.828571 -0.814286 -0.8 -0.785714 -0.771429 -0.757143 -0.742857 -0.728571 -0.714286 -0.7 -0.685714 -0.671429 -0.657143 -0.642857 -0.628571 -0.614286 -0.6 -0.585714 -0.571429 -0.557143 -0.542857 -0.528571 -0.514286 -0.5 -0.485714 -0.471429 -0.457143 -0.442857 -0.428571 -0.414286 -0.405839 -0.405839 -0.405839 -0.405839 -0.405839 -0.405839
  arc A152 (41.7843, -108.2568) -> (42.8106, -107.4297) centre (-2.0032, -52.8695) ccw
  spline S152 degree 5 poles (42.8106, -107.4297) (42.8193, -107.4359) (42.8425, -107.4523) (42.8803, -107.4791) (42.9329, -107.516) (43.0003, -107.563) (43.0741, -107.6138) (43.1481, -107.6644) (43.2225, -107.7146) (43.2971, -107.7646) (43.372, -107.8142) (43.4471, -107.8636) (43.5226, -107.9127) (43.5983, -107.9616) (43.6742, -108.0101) (43.7504, -108.0584) (43.8269, -108.1064) (43.9036, -108.1541) (43.9805, -108.2016) (44.0577, -108.2487) (44.1352, -108.2957) (44.2128, -108.3423) (44.2907, -108.3887) (44.3689, -108.4349) (44.4472, -108.4808) (44.5258, -108.5264) (44.6047, -108.5718) (44.6837, -108.6169) (44.763, -108.6618) (44.8425, -108.7064) (44.9222, -108.7508) (45.0021, -108.7949) (45.0822, -108.8388) (45.1625, -108.8825) (45.2431, -108.9259) (45.3238, -108.969) (45.4047, -109.012) (45.4859, -109.0546) (45.5672, -109.0971) (45.6488, -109.1393) (45.7305, -109.1813) (45.8125, -109.223) (45.8946, -109.2645) (45.9605, -109.2975) (46.0099, -109.3222) (46.043, -109.3386) (46.0595, -109.3468) knots 0.405839 0.405839 0.405839 0.405839 0.405839 0.405839 0.414286 0.428571 0.442857 0.457143 0.471429 0.485714 0.5 0.514286 0.528571 0.542857 0.557143 0.571429 0.585714 0.6 0.614286 0.628571 0.642857 0.657143 0.671429 0.685714 0.7 0.714286 0.728571 0.742857 0.757143 0.771429 0.785714 0.8 0.814286 0.828571 0.842857 0.857143 0.871429 0.885714 0.9 0.914286 0.928571 0.942857 0.957143 0.971429 0.985714 1 1 1 1 1 1
  arc A153 (46.0595, -109.3468) -> (47.0592, -108.4805) centre (-2.0032, -52.8695) ccw
  spline S153 degree 5 poles (47.0592, -108.4805) (47.0534, -108.463) (47.0419, -108.428) (47.0245, -108.3755) (47.0012, -108.3056) (46.9718, -108.2184) (46.9422, -108.1314) (46.9123, -108.0445) (46.8821, -107.9578) (46.8517, -107.8712) (46.821, -107.7848) (46.79, -107.6986) (46.7588, -107.6125) (46.7273, -107.5266) (46.6955, -107.4409) (46.6635, -107.3553) (46.6311, -107.27) (46.5986, -107.1848) (46.5657, -107.0997) (46.5326, -107.0149) (46.4991, -106.9302) (46.4654, -106.8457) (46.4314, -106.7615) (46.3972, -106.6774) (46.3626, -106.5934) (46.3278, -106.5097) (46.2926, -106.4262) (46.2572, -106.3429) (46.2215, -106.2597) (46.1855, -106.1768) (46.1491, -106.0941) (46.1125, -106.0116) (46.0756, -105.9293) (46.0383, -105.8472) (46.0008, -105.7653) (45.9629, -105.6837) (45.9247, -105.6023) (45.8862, -105.5211) (45.8474, -105.4401) (45.8082, -105.3594) (45.7687, -105.2789) (45.7289, -105.1987) (45.692, -105.1252) (45.663, -105.0679) (45.6419, -105.0266) (45.6289, -105.0013) (45.624, -104.9919) knots -1 -1 -1 -1 -1 -1 -0.985714 -0.971429 -0.957143 -0.942857 -0.928571 -0.914286 -0.9 -0.885714 -0.871429 -0.857143 -0.842857 -0.828571 -0.814286 -0.8 -0.785714 -0.771429 -0.757143 -0.742857 -0.728571 -0.714286 -0.7 -0.685714 -0.671429 -0.657143 -0.642857 -0.628571 -0.614286 -0.6 -0.585714 -0.571429 -0.557143 -0.542857 -0.528571 -0.514286 -0.5 -0.485714 -0.471429 -0.457143 -0.442857 -0.428571 -0.414286 -0.405839 -0.405839 -0.405839 -0.405839 -0.405839 -0.405839
  arc A154 (45.624, -104.9919) -> (46.5887, -104.0937) centre (-2.0032, -52.8695) ccw
  spline S154 degree 5 poles (46.5887, -104.0937) (46.5978, -104.0992) (46.6221, -104.114) (46.6617, -104.138) (46.7168, -104.1711) (46.7875, -104.2131) (46.8647, -104.2586) (46.9421, -104.3037) (47.0199, -104.3485) (47.0978, -104.393) (47.1761, -104.4372) (47.2546, -104.4811) (47.3333, -104.5247) (47.4123, -104.568) (47.4915, -104.611) (47.571, -104.6537) (47.6506, -104.6962) (47.7306, -104.7383) (47.8107, -104.7801) (47.8911, -104.8217) (47.9717, -104.863) (48.0525, -104.904) (48.1335, -104.9447) (48.2147, -104.9852) (48.2962, -105.0253) (48.3778, -105.0653) (48.4597, -105.1049) (48.5417, -105.1443) (48.624, -105.1834) (48.7065, -105.2222) (48.7891, -105.2608) (48.872, -105.2991) (48.955, -105.3372) (49.0383, -105.375) (49.1217, -105.4125) (49.2053, -105.4498) (49.2891, -105.4869) (49.3731, -105.5236) (49.4573, -105.5602) (49.5416, -105.5965) (49.6261, -105.6325) (49.7109, -105.6683) (49.7957, -105.7038) (49.8638, -105.7321) (49.9149, -105.7531) (49.949, -105.7671) (49.9661, -105.7741) knots 0.405839 0.405839 0.405839 0.405839 0.405839 0.405839 0.414286 0.428571 0.442857 0.457143 0.471429 0.485714 0.5 0.514286 0.528571 0.542857 0.557143 0.571429 0.585714 0.6 0.614286 0.628571 0.642857 0.657143 0.671429 0.685714 0.7 0.714286 0.728571 0.742857 0.757143 0.771429 0.785714 0.8 0.814286 0.828571 0.842857 0.857143 0.871429 0.885714 0.9 0.914286 0.928571 0.942857 0.957143 0.971429 0.985714 1 1 1 1 1 1
  arc A155 (49.9661, -105.7741) -> (50.9014, -104.8388) centre (-2.0032, -52.8695) ccw
  spline S155 degree 5 poles (50.9014, -104.8388) (50.8944, -104.8217) (50.8804, -104.7876) (50.8594, -104.7365) (50.8311, -104.6684) (50.7956, -104.5835) (50.7598, -104.4988) (50.7238, -104.4143) (50.6875, -104.33) (50.651, -104.2458) (50.6142, -104.1618) (50.5771, -104.078) (50.5398, -103.9944) (50.5023, -103.911) (50.4645, -103.8277) (50.4264, -103.7447) (50.3881, -103.6618) (50.3495, -103.5792) (50.3107, -103.4967) (50.2716, -103.4144) (50.2322, -103.3324) (50.1926, -103.2505) (50.1527, -103.1689) (50.1125, -103.0874) (50.072, -103.0062) (50.0313, -102.9252) (49.9903, -102.8444) (49.949, -102.7638) (49.9074, -102.6834) (49.8656, -102.6033) (49.8235, -102.5233) (49.781, -102.4437) (49.7383, -102.3642) (49.6953, -102.285) (49.652, -102.206) (49.6084, -102.1273) (49.5645, -102.0488) (49.5203, -101.9705) (49.4758, -101.8926) (49.431, -101.8148) (49.3859, -101.7374) (49.3404, -101.6602) (49.2984, -101.5895) (49.2653, -101.5344) (49.2413, -101.4948) (49.2265, -101.4705) (49.221, -101.4614) knots -1 -1 -1 -1 -1 -1 -0.985714 -0.971429 -0.957143 -0.942857 -0.928571 -0.914286 -0.9 -0.885714 -0.871429 -0.857143 -0.842857 -0.828571 -0.814286 -0.8 -0.785714 -0.771429 -0.757143 -0.742857 -0.728571 -0.714286 -0.7 -0.685714 -0.671429 -0.657143 -0.642857 -0.628571 -0.614286 -0.6 -0.585714 -0.571429 -0.557143 -0.542857 -0.528571 -0.514286 -0.5 -0.485714 -0.471429 -0.457143 -0.442857 -0.428571 -0.414286 -0.405839 -0.405839 -0.405839 -0.405839 -0.405839 -0.405839
  arc A156 (49.221, -101.4614) -> (50.1192, -100.4967) centre (-2.0032, -52.8695) ccw
  spline S156 degree 5 poles (50.1192, -100.4967) (50.1286, -100.5016) (50.1539, -100.5146) (50.1952, -100.5356) (50.2525, -100.5647) (50.326, -100.6016) (50.4062, -100.6414) (50.4867, -100.6809) (50.5674, -100.7201) (50.6484, -100.7589) (50.7296, -100.7974) (50.811, -100.8356) (50.8927, -100.8735) (50.9745, -100.911) (51.0566, -100.9483) (51.1389, -100.9852) (51.2214, -101.0218) (51.3041, -101.0582) (51.3871, -101.0942) (51.4702, -101.1299) (51.5535, -101.1653) (51.637, -101.2005) (51.7207, -101.2353) (51.8047, -101.2699) (51.8888, -101.3041) (51.9731, -101.3381) (52.0575, -101.3718) (52.1422, -101.4052) (52.227, -101.4384) (52.3121, -101.4712) (52.3973, -101.5038) (52.4826, -101.5361) (52.5682, -101.5682) (52.6539, -101.6) (52.7398, -101.6315) (52.8259, -101.6627) (52.9121, -101.6936) (52.9985, -101.7243) (53.0851, -101.7548) (53.1718, -101.785) (53.2587, -101.8149) (53.3457, -101.8445) (53.4329, -101.8739) (53.5028, -101.8972) (53.5553, -101.9146) (53.5903, -101.9261) (53.6078, -101.9319) knots 0.405839 0.405839 0.405839 0.405839 0.405839 0.405839 0.414286 0.428571 0.442857 0.457143 0.471429 0.485714 0.5 0.514286 0.528571 0.542857 0.557143 0.571429 0.585714 0.6 0.614286 0.628571 0.642857 0.657143 0.671429 0.685714 0.7 0.714286 0.728571 0.742857 0.757143 0.771429 0.785714 0.8 0.814286 0.828571 0.842857 0.857143 0.871429 0.885714 0.9 0.914286 0.928571 0.942857 0.957143 0.971429 0.985714 1 1 1 1 1 1
  arc A157 (53.6078, -101.9319) -> (54.4741, -100.9322) centre (-2.0032, -52.8695) ccw
  spline S157 degree 5 poles (54.4741, -100.9322) (54.4659, -100.9157) (54.4495, -100.8826) (54.4248, -100.8331) (54.3918, -100.7673) (54.3503, -100.6852) (54.3086, -100.6032) (54.2666, -100.5215) (54.2244, -100.4399) (54.1819, -100.3586) (54.1393, -100.2774) (54.0963, -100.1965) (54.0532, -100.1157) (54.0098, -100.0352) (53.9661, -99.9549) (53.9222, -99.8748) (53.8781, -99.7948) (53.8337, -99.7152) (53.7891, -99.6357) (53.7442, -99.5564) (53.6991, -99.4774) (53.6537, -99.3985) (53.6081, -99.3199) (53.5622, -99.2416) (53.516, -99.1634) (53.4696, -99.0855) (53.423, -99.0078) (53.3761, -98.9304) (53.3289, -98.8532) (53.2814, -98.7763) (53.2337, -98.6996) (53.1857, -98.6231) (53.1374, -98.5469) (53.0889, -98.4709) (53.04, -98.3953) (52.9909, -98.3198) (52.9416, -98.2447) (52.8919, -98.1698) (52.8419, -98.0952) (52.7917, -98.0208) (52.7411, -97.9468) (52.6903, -97.873) (52.6433, -97.8056) (52.6064, -97.753) (52.5796, -97.7151) (52.5632, -97.6919) (52.557, -97.6833) knots -1 -1 -1 -1 -1 -1 -0.985714 -0.971429 -0.957143 -0.942857 -0.928571 -0.914286 -0.9 -0.885714 -0.871429 -0.857143 -0.842857 -0.828571 -0.814286 -0.8 -0.785714 -0.771429 -0.757143 -0.742857 -0.728571 -0.714286 -0.7 -0.685714 -0.671429 -0.657143 -0.642857 -0.628571 -0.614286 -0.6 -0.585714 -0.571429 -0.557143 -0.542857 -0.528571 -0.514286 -0.5 -0.485714 -0.471429 -0.457143 -0.442857 -0.428571 -0.414286 -0.405839 -0.405839 -0.405839 -0.405839 -0.405839 -0.405839
  arc A158 (52.557, -97.6833) -> (53.3841, -96.657) centre (-2.0032, -52.8695) ccw